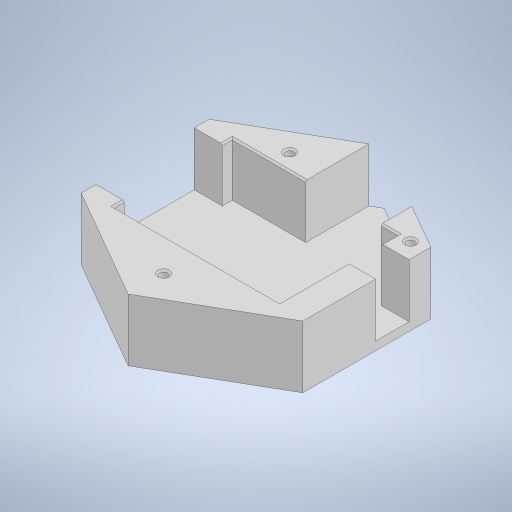
# Autodesk Inventor part: pi_case_bottom
Saved by Autodesk Inventor 2024 (Build 280153000, 153)
## iProperties
Created: 2024-03-18
Part Number: pi_case_bottom
Material: 일반
Document SubType Name: Modeling
Designer: SSAFY
Density: 1 g/cm^3
Appearance: 기본값
Author: SSAFY
Autodesk Inventor part; units mm, degrees
ref_plane "YZ Plane" through (0, 0, 0) normal (1, 0, 0) x (0, 1, 0)
ref_plane "XZ Plane" through (0, 0, 0) normal (0, 1, 0) x (-1, 0, 0)
ref_plane "XY Plane" through (0, 0, 0) normal (0, 0, 1) x (1, 0, 0)
sketch "스케치2" plane through (0, 0, 0) normal (0, 1, 0) x (-1, 0, 0)
  line L0 (0, -70.4) -> (-60.9682, -35.2)
  line L1 (-60.9682, -35.2) -> (-60.9682, 35.2)
  line L2 (-60.9682, 35.2) -> (0, 70.4)
  line L3 (0, 70.4) -> (60.9682, 35.2)
  line L4 (60.9682, 35.2) -> (60.9682, -35.2)
  line L5 (60.9682, -35.2) -> (0, -70.4)
  line L6 (60.9682, -35.2) -> (-60.9682, -35.2)
  line L7 (-60.9682, -35.2) -> (-60.9682, 35.2)
  line L8 (-60.9682, 35.2) -> (60.9682, 35.2)
  line L9 (60.9682, 35.2) -> (60.9682, -35.2)
  line L10 (60.9682, -35.2) -> (-60.9682, 35.2) construction
  line L11 (-60.9682, -35.2) -> (60.9682, 35.2) construction
  line L12 (0, 76.1735) -> (-65.9682, 38.0868)
  line L13 (-65.9682, 38.0868) -> (-65.9682, -38.0868)
  line L14 (-65.9682, -38.0868) -> (0, -76.1735)
  line L15 (0, -76.1735) -> (65.9682, -38.0868)
  line L16 (65.9682, -38.0868) -> (65.9682, 38.0868)
  line L17 (65.9682, 38.0868) -> (0, 76.1735)
  line L18 (49.325, -35.2) -> (-49.325, -35.2)
  line L19 (-49.325, -35.2) -> (-49.325, 35.2)
  line L20 (-49.325, 35.2) -> (49.325, 35.2)
  line L21 (49.325, 35.2) -> (49.325, -35.2)
  line L22 (49.325, -35.2) -> (-49.325, 35.2) construction
  line L23 (-49.325, -35.2) -> (49.325, 35.2) construction
  line L24 (49.325, 35.2) -> (65.9682, 35.2)
  line L25 (65.9682, 35.2) -> (65.9682, 29.2)
  line L26 (65.9682, 29.2) -> (49.325, 29.2)
  line L27 (49.325, 29.2) -> (49.325, 35.2)
  line L28 (49.325, -35.2) -> (65.9682, -35.2)
  line L29 (65.9682, -35.2) -> (65.9682, -29.2)
  line L30 (65.9682, -29.2) -> (49.325, -29.2)
  line L31 (49.325, -29.2) -> (49.325, -35.2)
  line L32 (5.675, -35.2) -> (5.675, -72.897)
  line L33 (-49.325, -25.2) -> (-65.9682, -25.2)
  line L34 (-65.9682, -25.2) -> (-65.9682, -5.2)
  line L35 (-65.9682, -5.2) -> (-49.325, -5.2)
  line L36 (-49.325, -5.2) -> (-49.325, -25.2)
  line L37 (-39.325, -35.2) -> (-39.325, -53.4692)
  point P0 (0, 0)
  point P1 (0, 0)
  dimension "d2" = 70.4
  dimension "d3" = 70.4
  dimension "d4" = 5
  dimension "d5" = 98.65
  dimension "d6" = 6
  dimension "d7" = 6
  dimension "d9" = 10
  dimension "d10" = 30
  dimension "d15" = 10
  dimension "d16" = 55
  constraints: 76 end point, 11 equal length, 10 point on line, 5 horizontal, 5 perpendicular, 4 midpoint, 2 vertical, 1 coincident, 18 other
  measures "d2" distance between parallel lines of L6 L8
  measures "d3" distance of L3.end L4.end
  measures "d4" distance between parallel lines of L2 L12
  measures "d5" distance between parallel lines of L21 L19
  measures "d6" distance between parallel lines of L28 L30
  measures "d7" distance between parallel lines of L26 L24
  measures "d9" distance between parallel lines of L6 L33
  measures "d10" distance between parallel lines of L6 L35
  measures "d15" distance between parallel lines of L37 L19
  measures "d16" distance between parallel lines of L32 L19
extrude "돌출1" add sketch "스케치2" along normal blind 32 contours L37 L14 L13 L33 L1 L0 | L0 L6 L37 | L32 L6 L5 | L5 L28 L16 L15 L32 | L1 L33 L19 L6 | L6 L21 L30 L4 | L4 L30 L16 L28 | L35 L13 L12 L17 L16 L24 L3 L2 L1 | L1 L8 L19 L35 | L26 L21 L8 L4 | L4 L24 L16 L26 | L2 L3 L8
sketch "스케치3" plane through (0, 0, 0) normal (0, 1, 0) x (-1, 0, 0)
  line L0 (0, 76.1735) -> (-65.9682, 38.0868) construction
  line L1 (0, 76.1735) -> (65.9682, 38.0868)
  line L2 (65.9682, 38.0868) -> (65.9682, -38.0868)
  line L3 (65.9682, -38.0868) -> (0, -76.1735)
  line L4 (0, -76.1735) -> (-65.9682, -38.0868)
  line L5 (-65.9682, -38.0868) -> (-65.9682, 38.0868)
  line L6 (-65.9682, 38.0868) -> (0, 76.1735)
  point P0 (0, 0)
  point P1 (0, 0)
  constraints: 12 end point, 1 coincident, 13 other
extrude "돌출2" add sketch "스케치3" against normal blind 5
sketch "스케치4" plane through (0, 32, 0) normal (0, 1, 0) x (1, 0, 0)
  circle A0 centre (0, -55) radius 2.5
  circle A1 centre (-25, 45) radius 2.5
  circle A2 centre (57, 35) radius 2.5
  point P0 (0, 0)
  dimension "d17" = 5
  dimension "d18" = 55
  dimension "d19" = 5
  dimension "d20" = 45
  dimension "d21" = 25
  dimension "d22" = 5
  dimension "d23" = 57
  dimension "d24" = 35
  constraints: 3 centre point
  measures "d17" diameter of A0
  measures "d18" distance of A0.centre point (0, 0)
  measures "d19" diameter of A1
  measures "d20" vertical distance of point (0, 0) A1.centre
  measures "d21" horizontal distance of point (0, 0) A1.centre
  measures "d22" diameter of A2
  measures "d23" horizontal distance of A2.centre point (0, 0)
  measures "d24" vertical distance of point (0, 0) A2.centre
extrude "돌출3" cut sketch "스케치4" against normal blind 5
chamfer "모따기1" distance 1 angle 45 10 edges at (-2.5, 32, 55) (-27.5, 32, -45) (54.5, 32, -35) (-27.5, 32, -35.2) (-49.325, 32, -32.2) (-49.325, 32, 32.2) (0, 32, 35.2) (44.325, 32, -35.2) (49.325, 32, -30.2) (49.325, 32, 15)
equation "\"d3\" = d2"
